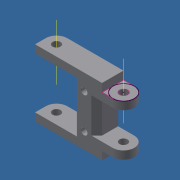
# Autodesk Inventor part: FingerPartB
Saved by Autodesk Inventor 2014 SP2 (Build 180246200, 246)
## iProperties
Created: 2014-12-28
Part Number: FingerPartB
Material: Generisch
Document SubType Name: Modeling
Designer: 4ndreas
Density: 1 g/cm^3
Appearance: Vorgabe
Mass: 2.87681 g
Surface Area: 21.8978 cm^2
Volume: 2.87681 cm^3
Author: 4ndreas
Autodesk Inventor part; units mm, degrees
ref_plane "YZ Plane" through (0, 0, 0) normal (1, 0, 0) x (0, 1, 0)
ref_plane "XZ Plane" through (0, 0, 0) normal (0, 1, 0) x (-1, 0, 0)
ref_plane "XY Plane" through (0, 0, 0) normal (0, 0, 1) x (1, 0, 0)
sketch "Skizze1" plane through (0, 0, 0) normal (0, 0, 1) x (1, 0, 0)
  circle A0 centre (0, 0) radius 4 construction
  circle A1 centre (-25, 0) radius 4 construction
  line L0 (-25, 0) -> (0, 0) construction
  line L1 (-29, 0) -> (-29, -4)
  line L2 (-29, -4) -> (0, -4)
  line L3 (0, 4) -> (-25, 4)
  arc A2 (-25, 4) -> (-29, 0) centre (-25, 0) ccw
  arc A3 (0, -4) -> (0, 4) centre (0, 0) ccw
  dimension "d0" = 8
  dimension "d1" = 25
  constraints: 8 end point, 6 point on circle, 3 centre point, 3 coincident, 3 horizontal, 2 tangent, 1 horizontal alignment, 1 perpendicular, 1 vertical, 3 other
  measures "d1" distance of L0.start L0.end
extrude "Extrusion1" add sketch "Skizze1" along normal blind 3
sketch "Skizze2" plane through (0, 0, 0) normal (0, 0, -1) x (-1, 0, 0)
  arc A0 (29, 0) -> (25, 4) centre (25, 0) ccw projected
  line L0 (0, 4) -> (25, 4) projected
  arc A1 (0, 4) -> (0, -4) centre (0, 0) ccw projected
  line L1 (29, -4) -> (0, -4) projected
  line L2 (6, 4) -> (19, 4)
  line L3 (19, 4) -> (19, -4)
  line L4 (19, -4) -> (6, -4)
  line L5 (6, -4) -> (6, 4)
  dimension "d4" = 4
  dimension "d5" = 6
  dimension "d6" = 6
  constraints: 8 end point, 2 parallel, 2 point on line, 1 horizontal, 1 perpendicular
  measures "d4" radius of A1
  measures "d5" distance from line of A1.centre L5
  measures "d6" distance from line of L3 A0.centre
extrude "Extrusion2" add sketch "Skizze2" along normal blind 9.5 contours L0 L3 L1 L5
sketch "Skizze3" plane through (0, 0, 0) normal (0, 0, -1) x (-1, 0, 0)
  line L0 (6, -4) -> (6, 4) projected
  line L1 (0, 4) -> (6, 4) projected
  arc A0 (0, 4) -> (0, -4) centre (0, 0) ccw projected
  line L2 (6, -4) -> (0, -4) projected
extrude "Extrusion3" add sketch "Skizze3" along normal blind 3
sketch "Skizze4" plane through (0, 0, 3) normal (0, 0, 1) x (1, 0, 0)
  line L0 (-6, 4) -> (-6, -4) projected
  line L1 (-6, 4) -> (0, 4) projected
  arc A0 (0, -4) -> (0, 4) centre (0, 0) ccw projected
  line L2 (0, -4) -> (-6, -4) projected
extrude "Extrusion4" cut sketch "Skizze4" against normal blind 3
mirror "Spiegeln1" about plane through (-12.5, 0, -9.5) normal (0, 0, -1)
sketch "Skizze5" plane through (0, 0, 0) normal (0, 0, -1) x (-1, 0, 0)
  line L0 (19, 4) -> (19, -4) projected
  line L1 (19, 4) -> (25, 4) projected
  line L2 (19, 4) -> (13.3983, -4)
  line L3 (13.3983, -4) -> (19, -4)
  point P0 (0, 0)
  dimension "d13" = 35
  constraints: 4 end point, 1 parallel
  measures "d13" angle of L0 L2
extrude "Extrusion5" cut sketch "Skizze5" along normal up to surface (19 mm away)
sketch "Skizze6" plane through (0, 0, 3) normal (0, 0, 1) x (1, 0, 0)
  arc A0 (-25, 4) -> (-29, 0) centre (-25, 0) ccw projected
  point P0 (0, 0)
hole "Bohrung1" at (-25, 0, 3) direction (0, 0, -1) diameter 3 end through all
hole "Bohrung2" at (0, 0, 3) direction (0, 0, -1) diameter 3 end through all
sketch "Skizze7" plane through (-6, -4, 3) normal (1, 0, 0) x (0, 0, -1)
  line L0 (0, 0) -> (0, 8) projected
  line L1 (3, 0) -> (0, 0) projected
  line L2 (3, 0) -> (3, 8) projected
  line L3 (0, 8) -> (3, 8) projected
  line L4 (22, 0) -> (25, 0) projected
  line L5 (25, 0) -> (25, 8) projected
  line L6 (25, 8) -> (22, 8) projected
  line L7 (22, 0) -> (22, 8) projected
  line L8 (22, 0) -> (25, 0) projected
  point P0 (3, 4)
extrude "Extrusion6" add sketch "Skizze7" along normal blind 2
chamfer "Fase1" distance 2 angle 45 1 edges at (-6, -4, -9.5)
sketch "Skizze8" plane through (-25, 4, 3) normal (0, 1, 0) x (1, 0, 0)
  line L0 (17, 19) -> (25, 19) projected
  line L1 (17, 6) -> (17, 19) projected
  line L2 (25, 6) -> (17, 6) projected
  line L3 (25, 6) -> (25, 3) projected
  line L4 (25, 3) -> (21, 3) projected
  line L5 (21, 0) -> (21, 3) projected
  line L6 (-4, 0) -> (21, 0) projected
  line L7 (-4, 3) -> (-4, 0) projected
  line L8 (-4, 3) -> (11.6017, 3) projected
  line L9 (11.6017, 3) -> (11.6017, 22) projected
  line L10 (11.6017, 22) -> (-4, 22) projected
  line L11 (-4, 22) -> (-4, 25) projected
  line L12 (-4, 25) -> (21, 25) projected
  line L13 (21, 22) -> (21, 25) projected
  line L14 (25, 22) -> (21, 22) projected
  line L15 (25, 19) -> (25, 22) projected
  line L16 (17, 19) -> (11.6017, 19)
  line L17 (17, 6) -> (11.6017, 6)
  point P0 (14.3008, 19)
  point P1 (14.3008, 6)
  constraints: 4 end point, 2 midpoint, 2 perpendicular, 2 point on line
hole "Bohrung3" at (-10.6992, 4, -16) at (-10.6992, 4, -3) direction (0, -1, 0) diameter 2.5 end through all countersink diameter 4 countersink angle 90
sketch "Skizze9" plane through (0, 0, 0) normal (0, 0, 1) x (1, 0, 0)
  line L0 (-4, 4) -> (-4, -4) projected
  line L1 (0, -4) -> (-4, -4) projected
  arc A0 (0, -4) -> (0, 4) centre (0, 0) ccw projected
  line L2 (-4, 4) -> (0, 4) projected
  circle A1 centre (0, 0) radius 1.5 projected
  circle A2 centre (0, 0) radius 4
  constraints: 1 coincident, 1 vertical alignment, 2 other
equation "\"d0\" = Finger_diameter"
equation "\"d1\" = FingerLaenge_B"
equation "\"d2\" = FingerWall"
equation "\"d5\" = 1.5 * d4"
equation "\"d6\" = d5"
equation "\"d7\" = -0.5 * FingerWall + 0.5 * Finger_width"
equation "\"d9\" = FingerWall"
equation "\"d11\" = FingerWall"
equation "\"d29\" = bearingHole"
equation "\"FingerLaenge_B\" = 25"
equation "\"Hebel_B\" = 25"
equation "\"Finger_width\" = 22"
equation "\"Finger_diameter\" = 8"
equation "\"FingerWall\" = 3"
equation "\"Hebel_basis_2\" = 15"
equation "\"Join_width\" = 3"
equation "\"bearingHole\" = 3"
equation "\"bearingWall\" = 4"
equation "\"support_D\" = 0.25"
